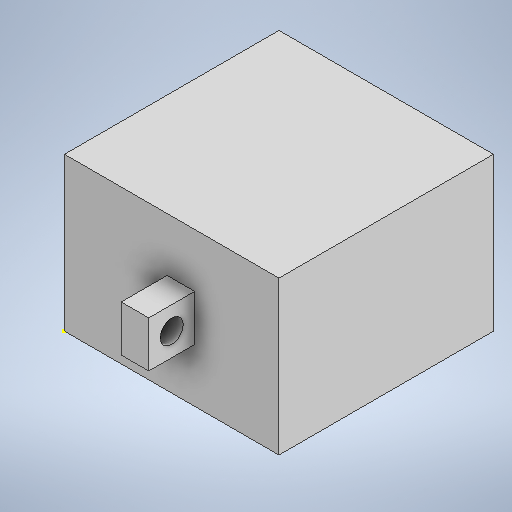
# Autodesk Inventor part: Balancin
Saved by Autodesk Inventor 2025.2 (Build 292293000, 293)
## iProperties
Created: 2026-09-08
Part Number: Balancin
Material: Generic
Document SubType Name: Sheet Metal
Designer: dguar
Density: 1 g/cm^3
Sheet Metal Rule: Default_mm
Appearance: Default
Author: dguar
Autodesk Inventor part; units mm, degrees
ref_plane "YZ Plane" through (0, 0, 0) normal (1, 0, 0) x (0, 1, 0)
ref_plane "XZ Plane" through (0, 0, 0) normal (0, 1, 0) x (-1, 0, 0)
ref_plane "XY Plane" through (0, 0, 0) normal (0, 0, 1) x (1, 0, 0)
sketch "Sketch1" plane through (0, 0, 0) normal (1, 0, 0) x (0, 1, 0)
  point P0 (0, 0)
sketch "Sketch2" plane through (0, 0, 0) normal (0, 1, 0) x (-1, 0, 0)
  line L0 (0, 0) -> (-140, 0)
  line L1 (-140, 0) -> (-140, -140)
  line L2 (-140, -140) -> (0, -140)
  line L3 (0, -140) -> (0, 0)
  dimension "d0" = 140
  dimension "d1" = 140
  constraints: 8 end point, 2 parallel, 1 horizontal, 1 perpendicular
  measures "d0" distance of L2.end L1.end
  measures "d1" distance of L1.end L0.end
extrude "Extrusion1" add sketch "Sketch2" along normal blind 100
sketch "Sketch3" plane through (0, 0, 0) normal (0, 0, 1) x (1, 0, 0)
  line L0 (140, 100) -> (0, 100) projected
  line L1 (140, 0) -> (140, 100) projected
  line L2 (140, 0) -> (0, 0) projected
  line L3 (70, 35) -> (73, 35)
  line L4 (73, 35) -> (67, 35)
  line L5 (67, 35) -> (67, 65)
  line L6 (67, 65) -> (73, 65)
  line L7 (73, 65) -> (73, 35)
  constraints: 10 end point, 3 perpendicular, 1 point on line
extrude "Extrusion2" add sketch "Sketch3" along normal blind 30
sketch "Sketch4" plane through (73, 35, 0) normal (1, 0, 0) x (0, 0, -1)
  line L0 (0, -35) -> (0, 65) projected
  circle A0 centre (-15.0175, 14.9912) radius 7.5
  point P0 (-30, 30)
  dimension "d10" = 15
  constraints: 1 centre point
  measures "d10" diameter of A0
extrude "Extrusion3" cut sketch "Sketch4" against normal blind 30
sketch "Sketch5" plane through (73, 35, 0) normal (1, 0, 0) x (0, 0, -1)
  line L0 (0, 30) -> (0, 0) projected
  line L1 (-30, 30) -> (0, 30)
  line L2 (0, 30) -> (0, 0)
  line L3 (0, 0) -> (-30, 0)
  line L4 (-30, 0) -> (-30, 30)
  circle A0 centre (-15, 15) radius 7.5088
  point P0 (0, -35)
  constraints: 8 end point, 2 parallel, 1 centre point, 1 horizontal, 1 perpendicular
extrude "Extrusion4" add sketch "Sketch5" along normal blind 12
equation "\"BendRadius\" = Thickness"
equation "\"BendReliefWidth\" = Thickness"
equation "\"BendReliefDepth\" = 0.5 * Thickness"
equation "\"CornerReliefSize\" = 4 * Thickness"
equation "\"MinimumRemnant\" = 2 * Thickness"
equation "\"TransitionRadius\" = BendRadius"
equation "\"JacobiRadiusSize\" = BendRadius"
equation "\"GapSize\" = Thickness"
equation "\"Thickness\" = 0.5"
body "Solid1"
